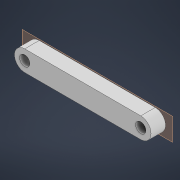
# Autodesk Inventor part: 2HoleLinkage
Saved by Autodesk Inventor 2021 (Build 250183000, 183)
## iProperties
Created: 2021-01-28
Part Number: 2HoleLinkage
Material: Generic
Document SubType Name: Modeling
Designer: argon
Density: 1 g/cm^3
Appearance: Default
Author: argon
Autodesk Inventor part; units mm, degrees
ref_plane "YZ Plane" through (0, 0, 0) normal (1, 0, 0) x (0, 1, 0)
ref_plane "XZ Plane" through (0, 0, 0) normal (0, 1, 0) x (-1, 0, 0)
sketch "Sketch1" plane through (0, 0, 0) normal (0, 0, 1) x (1, 0, 0)
  circle A0 centre (-24, 0) radius 2.125
  circle A1 centre (24, 0) radius 2.125
  line L0 (-24, 0) -> (0, 0) construction
  line L1 (0, 0) -> (24, 0) construction
  line L2 (-24, 4.25) -> (24, 4.25)
  line L3 (-24, -4.25) -> (24, -4.25)
  line L4 (0, 4.25) -> (0, -4.25) construction
  arc A2 (-24, 4.25) -> (-24, -4.25) centre (-24, 0) ccw
  arc A3 (24, -4.25) -> (24, 4.25) centre (24, 0) ccw
  point P0 (-24, -2.125)
  dimension "d0" = 4.25
  dimension "d1" = 2.125
  dimension "d2" = 24
  constraints: 10 end point, 4 point on circle, 3 centre point, 3 coincident, 3 horizontal, 3 midpoint, 3 vertical alignment, 2 equal length, 1 collinear, 1 vertical, 3 other
  measures "d1" distance of L3.start point (-24, -2.125)
  measures "d2" distance of L0.start L0.end
extrude "Extrusion1" add sketch "Sketch1" along normal blind 6
body "Solid1"
